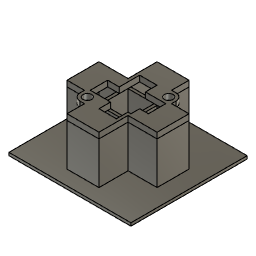
Button+Holder+Rev+3 (Autodesk Fusion 360 design; units mm, degrees)
Autodesk Fusion 360 part; units mm, degrees
note: some values were not read from the file. Set by a fixed rule: which sketch regions a step uses.
sketch "Button Face" plane through (0, 0, 0) normal (0, 0, 1) x (1, 0, 0)
  line L0 (2, 4) -> (44, 4)
  line L1 (44, 4) -> (44, 44)
  line L2 (44, 44) -> (2, 44)
  line L3 (2, 44) -> (2, 4)
  line L4 (7, 30) -> (18, 30)
  line L5 (18, 30) -> (18, 19)
  line L6 (18, 19) -> (7, 19)
  line L7 (7, 19) -> (7, 30)
  line L8 (17, 29) -> (28, 29)
  line L9 (28, 29) -> (28, 40)
  line L10 (28, 40) -> (17, 40)
  line L11 (17, 40) -> (17, 29)
  line L12 (27, 30) -> (38, 30)
  line L13 (38, 30) -> (38, 19)
  line L14 (38, 19) -> (27, 19)
  line L15 (27, 19) -> (27, 30)
  line L16 (17, 20) -> (28, 20)
  line L17 (28, 20) -> (28, 9)
  line L18 (28, 9) -> (17, 9)
  line L19 (17, 9) -> (17, 20)
  line L20 (28, 29) -> (37, 29)
  line L21 (37, 29) -> (37, 20)
  line L22 (37, 20) -> (28, 20)
  line L23 (28, 20) -> (28, 29)
  line L24 (17, 29) -> (8, 29)
  line L25 (8, 29) -> (8, 20)
  line L26 (8, 20) -> (17, 20)
  line L27 (17, 20) -> (17, 29)
  line L28 (18, 19) -> (27, 19)
  line L29 (27, 19) -> (27, 10)
  line L30 (27, 10) -> (18, 10)
  line L31 (18, 10) -> (18, 19)
  line L32 (18, 30) -> (27, 30)
  line L33 (27, 30) -> (27, 39)
  line L34 (27, 39) -> (18, 39)
  line L35 (18, 39) -> (18, 30)
  circle A0 centre (22.5, 14.5) radius 3.6
  circle A1 centre (32.5, 24.5) radius 3.6
  circle A2 centre (22.5, 34.5) radius 3.6
  circle A3 centre (12.5, 24.5) radius 3.6
  circle A4 centre (29.5, 31.5) radius 1.5
  circle A5 centre (29.5, 31.5) radius 2.5
  line L36 (29.5, 34) -> (28, 34)
  line L37 (28, 34) -> (28, 33.5)
  line L38 (28, 33.5) -> (29.5, 33.5)
  line L39 (29.5, 33.5) -> (29.5, 34)
  line L40 (32, 31.5) -> (31.5, 31.5)
  line L41 (31.5, 31.5) -> (31.5, 30)
  line L42 (31.5, 30) -> (32, 30)
  line L43 (32, 30) -> (32, 31.5)
  circle A6 centre (15.5, 17.5) radius 1.5
  circle A7 centre (15.5, 17.5) radius 2.5
  line L44 (15.5, 15) -> (17, 15)
  line L45 (17, 15) -> (17, 15.5)
  line L46 (17, 15.5) -> (15.5, 15.5)
  line L47 (15.5, 15.5) -> (15.5, 15)
  line L48 (13, 17.5) -> (13.5, 17.5)
  line L49 (13.5, 17.5) -> (13.5, 19)
  line L50 (13.5, 19) -> (13, 19)
  line L51 (13, 19) -> (13, 17.5)
  dimension "d3" = 11
  dimension "d4" = 11
  dimension "d5" = 11
  dimension "d6" = 11
  dimension "d7" = 11
  dimension "d8" = 11
  dimension "d9" = 11
  dimension "d10" = 11
  dimension "d11" = 1
  dimension "d12" = 1
  dimension "d13" = 1
  dimension "d14" = 1
  dimension "d15" = 1
  dimension "d16" = 1
  dimension "d17" = 9
  dimension "d18" = 9
  dimension "d19" = 9
  dimension "d20" = 9
  dimension "d21" = 9
  dimension "d22" = 9
  dimension "d23" = 9
  dimension "d24" = 9
  dimension "d25" = 7.2
  dimension "d26" = 4.5
  dimension "d27" = 4.5
  dimension "d28" = 7.2
  dimension "d29" = 7.2
  dimension "d30" = 7.2
  dimension "d31" = 4.5
  dimension "d32" = 4.5
  dimension "d33" = 4.5
  dimension "d34" = 4.5
  dimension "d35" = 4.5
  dimension "d36" = 4.5
  dimension "d38" = 3
  dimension "d39" = 1.5
  dimension "d40" = 1.5
  dimension "d41" = 5
  dimension "d42" = 3
  dimension "d43" = 1.5
  dimension "d44" = 1.5
  dimension "d45" = 5
  constraint horizontal L0
  constraint vertical L1
  constraint horizontal L2
  constraint vertical L3
  constraint horizontal L4
  constraint vertical L5
  constraint horizontal L6
  constraint vertical L7
  constraint horizontal L8
  constraint vertical L9
  constraint horizontal L10
  constraint vertical L11
  constraint horizontal L12
  constraint vertical L13
  constraint horizontal L14
  constraint vertical L15
  constraint horizontal L16
  constraint vertical L17
  constraint horizontal L18
  constraint vertical L19
  constraint horizontal L20
  constraint vertical L21
  constraint horizontal L22
  constraint vertical L23
  constraint horizontal L24
  constraint vertical L25
  constraint horizontal L26
  constraint vertical L27
  constraint horizontal L28
  constraint vertical L29
  constraint horizontal L30
  constraint vertical L31
  constraint horizontal L32
  constraint vertical L33
  constraint horizontal L34
  constraint vertical L35
  constraint concentric A4 A5
  constraint horizontal L36
  constraint vertical L37
  constraint horizontal L38
  constraint vertical L39
  constraint coincident A5 L37.end
  constraint coincident L9 L37.end
  constraint coincident A5 L36.start
  constraint horizontal L40
  constraint vertical L41
  constraint horizontal L42
  constraint vertical L43
  constraint coincident A5 L41.end
  constraint coincident L12 L41.end
  constraint coincident A5 L40.start
  constraint concentric A6 A7
  constraint horizontal L44
  constraint vertical L45
  constraint horizontal L46
  constraint vertical L47
  constraint coincident A7 L45.end
  constraint coincident L19 L45.end
  constraint coincident A7 L44.start
  constraint horizontal L48
  constraint vertical L49
  constraint horizontal L50
  constraint vertical L51
  constraint coincident A7 L49.end
  constraint coincident L6 L49.end
  constraint coincident A7 L48.start
  measures "d3" distance of L4.start L4.end
  measures "d4" distance of L4.start L6.end
  measures "d5" distance of L8.start L8.end
  measures "d6" distance of L8.start L10.end
  measures "d7" distance of L12.start L12.end
  measures "d8" distance of L12.start L14.end
  measures "d9" distance of L16.start L16.end
  measures "d10" distance of L16.start L18.end
  measures "d11" distance of L15 L17
  measures "d12" distance of L14 L16
  measures "d13" distance of L5 L19
  measures "d14" distance of L6 L16
  measures "d15" distance of L9 L15
  measures "d16" distance of L8 L12
  measures "d17" distance of L8.end L20.end
  measures "d18" distance of L8.end L16.end
  measures "d19" distance of L8.start L24.end
  measures "d20" distance of L8.start L16.start
  measures "d21" distance of L5.end L14.end
  measures "d22" distance of L5.end L30.end
  measures "d23" distance of L4.end L12.start
  measures "d24" distance of L4.end L34.end
  measures "d25" diameter of A0
  measures "d26" distance of L31 A0.centre
  measures "d27" distance of L28 A0.centre
  measures "d28" diameter of A1
  measures "d29" diameter of A2
  measures "d30" diameter of A3
  measures "d31" distance of L24 A3.centre
  measures "d32" distance of L25 A3.centre
  measures "d33" distance of L35 A2.centre
  measures "d34" distance of L34 A2.centre
  measures "d35" distance of L23 A1.centre
  measures "d36" distance of L20 A1.centre
  measures "d38" diameter of A4
  measures "d39" distance of L9 A4.centre
  measures "d40" distance of L12 A4.centre
  measures "d41" diameter of A5
  measures "d42" diameter of A6
  measures "d43" distance of L19 A6.centre
  measures "d44" distance of L6 A6.centre
  measures "d45" diameter of A7
extrude "Extrude1" add sketch "Button Face" along normal blind 1 contours L0 L1 L2 L3 | L5 L8 L15 L16 makes body 1 at (36.6667, 10.6667, 0) makes body 2 at (21, 26, 0)
extrude "Extrude2" add sketch "Button Face" along normal blind 15.5 contours L4 L6 L7 L11 L24 L25 L26 A7 L50 | L4 L9 L10 L11 L33 L34 L35 A5 L37 | L4 L5 L8 L11 | L5 L8 L15 L32 | L5 L8 L16 L27 | L6 A7 L50 L51 | L12 L33 A5 | L8 L9 L12 L15 A5 | L5 L6 L16 L19 A7 | L19 L26 A7 | L6 L19 A7 | A7 L48 L49 | L6 L19 A6 A7 L46 L47 L48 L49 | L5 L15 L16 L28 | L8 L15 L16 L23 | L9 L12 A5 | L9 L12 A5 | L9 A5 L36 L37 | L6 L19 A7 | L6 L19 A6 | A7 L46 L47 | L19 A7 L44 L45 | L6 L31 A7 | L14 L15 L16 L17 | L9 L20 A5 | L9 L12 A5 | L9 L12 A4 | L9 L12 A4 A5 L38 L39 L40 L41 | A5 L38 L39 | L6 L19 A7 | L14 L17 L18 L19 L29 L30 L31 A7 L45 | L12 L13 L14 L17 L20 L21 L22 A5 L42 | L12 A5 L42 L43 | A5 L40 L41 bodies 1 2
extrude "Extrude3" add sketch "Button Face" along normal blind 1 contours A6 | A4 bodies 1
extrude "Extrude4" add sketch "Button Face" along normal blind 6.5 contours L32 L33 L34 L35 | L24 L25 L26 L27 | L28 L29 L30 L31 | L20 L21 L22 L23 bodies 1
sketch "Button Back" plane through (0, 0, 15.5) normal (0, 0, 1) x (-1, 0, 0)
  line L0 (-27, -10) -> (-18, -10)
  line L1 (-18, -10) -> (-18, -19)
  line L2 (-18, -19) -> (-27, -19)
  line L3 (-27, -19) -> (-27, -10)
  circle A0 centre (-15.5, -17.5) radius 1.5
  line L4 (-18, -20) -> (-18, -29)
  line L5 (-18, -29) -> (-27, -29)
  line L6 (-27, -29) -> (-27, -20)
  line L7 (-27, -20) -> (-18, -20)
  line L8 (-37, -20) -> (-28, -20)
  line L9 (-28, -20) -> (-28, -29)
  line L10 (-28, -29) -> (-37, -29)
  line L11 (-37, -29) -> (-37, -20)
  circle A1 centre (-29.5, -31.5) radius 1.5
  line L12 (-18, -30) -> (-18, -39)
  line L13 (-18, -39) -> (-27, -39)
  line L14 (-27, -39) -> (-27, -30)
  line L15 (-27, -30) -> (-18, -30)
  line L16 (-17, -29) -> (-17, -20)
  line L17 (-17, -20) -> (-8, -20)
  line L18 (-8, -20) -> (-8, -29)
  line L19 (-8, -29) -> (-17, -29)
  line L20 (-7, -19) -> (-13, -19)
  line L21 (-13, -19) -> (-13, -17.5)
  arc A2 (-13, -17.5) -> (-15.5, -15) centre (-15.5, -17.5) ccw
  line L22 (-15.5, -15) -> (-17, -15)
  line L23 (-17, -15) -> (-17, -9)
  line L24 (-17, -9) -> (-28, -9)
  line L25 (-28, -9) -> (-28, -19)
  line L26 (-28, -19) -> (-38, -19)
  line L27 (-38, -19) -> (-38, -30)
  line L28 (-38, -30) -> (-32, -30)
  line L29 (-32, -30) -> (-32, -31.5)
  arc A3 (-32, -31.5) -> (-29.5, -34) centre (-29.5, -31.5) ccw
  line L30 (-29.5, -34) -> (-28, -34)
  line L31 (-28, -34) -> (-28, -40)
  line L32 (-28, -40) -> (-17, -40)
  line L33 (-17, -40) -> (-17, -30)
  line L34 (-17, -30) -> (-7, -30)
  line L35 (-7, -30) -> (-7, -19)
  line L36 (-8, -29) -> (-17, -29)
  line L37 (-17, -29) -> (-17, -20)
  line L38 (-17, -20) -> (-8, -20)
  line L39 (-8, -20) -> (-8, -29)
  line L40 (-18, -19) -> (-27, -19)
  line L41 (-27, -19) -> (-27, -10)
  line L42 (-27, -10) -> (-18, -10)
  line L43 (-18, -10) -> (-18, -19)
  line L44 (-28, -20) -> (-37, -20)
  line L45 (-37, -20) -> (-37, -29)
  line L46 (-37, -29) -> (-28, -29)
  line L47 (-28, -29) -> (-28, -20)
  line L48 (-27, -30) -> (-18, -30)
  line L49 (-18, -30) -> (-18, -39)
  line L50 (-18, -39) -> (-27, -39)
  line L51 (-27, -39) -> (-27, -30)
  line L52 (-27, -19) -> (-21, -19)
  line L53 (-21, -19) -> (-21, -16)
  line L54 (-21, -16) -> (-27, -16)
  line L55 (-27, -16) -> (-27, -19)
  line L56 (-28, -29) -> (-31, -29)
  line L57 (-31, -29) -> (-31, -23)
  line L58 (-31, -23) -> (-28, -23)
  line L59 (-28, -23) -> (-28, -29)
  line L60 (-18, -30) -> (-24, -30)
  line L61 (-24, -30) -> (-24, -33)
  line L62 (-24, -33) -> (-18, -33)
  line L63 (-18, -33) -> (-18, -30)
  line L64 (-17, -20) -> (-14, -20)
  line L65 (-14, -20) -> (-14, -26)
  line L66 (-14, -26) -> (-17, -26)
  line L67 (-17, -26) -> (-17, -20)
  dimension "d66" = 6
  dimension "d67" = 3
  dimension "d68" = 3
  dimension "d69" = 6
  dimension "d70" = 6
  dimension "d71" = 3
  dimension "d72" = 3
  dimension "d73" = 6
  constraint horizontal L36
  constraint vertical L37
  constraint horizontal L38
  constraint vertical L39
  constraint coincident L16.end L17.start
  constraint coincident L18.end L19.start
  constraint horizontal L40
  constraint vertical L41
  constraint horizontal L42
  constraint vertical L43
  constraint coincident L0.start L3.end
  constraint coincident L1.end L2.start
  constraint horizontal L44
  constraint vertical L45
  constraint horizontal L46
  constraint vertical L47
  constraint coincident L10.end L11.start
  constraint coincident L8.end L9.start
  constraint horizontal L48
  constraint vertical L49
  constraint horizontal L50
  constraint vertical L51
  constraint coincident L12.end L13.start
  constraint coincident L14.end L15.start
  constraint horizontal L52
  constraint vertical L53
  constraint horizontal L54
  constraint vertical L55
  constraint coincident L2.end L3.start
  constraint horizontal L56
  constraint vertical L57
  constraint horizontal L58
  constraint vertical L59
  constraint coincident L9.end L10.start
  constraint horizontal L60
  constraint vertical L61
  constraint horizontal L62
  constraint vertical L63
  constraint coincident L12.start L15.end
  constraint horizontal L64
  constraint vertical L65
  constraint horizontal L66
  constraint vertical L67
  measures "d66" distance of L2.end L52.end
  measures "d67" distance of L2.end L54.end
  measures "d68" distance of L9.end L56.end
  measures "d69" distance of L9.end L58.end
  measures "d70" distance of L12.start L60.end
  measures "d71" distance of L12.start L62.end
  measures "d72" distance of L16.end L64.end
  measures "d73" distance of L16.end L66.end
extrude "Extrude5" add sketch "Button Back" along normal blind 1 separate body contours L0 L1 L2 L3 L40 L41 L42 L43 L53 L54 | L8 L9 L10 L11 L44 L45 L46 L47 L57 L58 | L12 L13 L14 L15 L48 L49 L50 L51 L61 L62 | L16 L17 L18 L19 L36 L37 L38 L39 L65 L66 | L20 L21 A2 L22 L23 L24 L25 L26 L27 L28 L29 A3 L30 L31 L32 L33 L34 L35 makes body 3
sketch "Back Wire" plane through (0, 0, 16.5) normal (0, 0, 1) x (-1, 0, 0)
  line L0 (-17, -26) -> (-17, -20)
  line L1 (-18, -30) -> (-18, -33)
  line L2 (-24, -30) -> (-18, -30)
  circle A0 centre (-15.5, -17.5) radius 1.5
  line L3 (-28, -23) -> (-28, -29)
  circle A1 centre (-29.5, -31.5) radius 1.5
  line L4 (-27, -29) -> (-27, -20)
  line L5 (-27, -20) -> (-18, -20)
  line L6 (-18, -20) -> (-18, -29)
  line L7 (-18, -29) -> (-27, -29)
  line L8 (-27, -19) -> (-27, -16)
  line L9 (-21, -19) -> (-27, -19)
  line L10 (-7, -30) -> (-7, -19)
  line L11 (-7, -19) -> (-13, -19)
  line L12 (-13, -19) -> (-13, -17.5)
  arc A2 (-13, -17.5) -> (-15.5, -15) centre (-15.5, -17.5) ccw
  line L13 (-15.5, -15) -> (-17, -15)
  line L14 (-17, -15) -> (-17, -9)
  line L15 (-17, -9) -> (-28, -9)
  line L16 (-28, -9) -> (-28, -19)
  line L17 (-28, -19) -> (-38, -19)
  line L18 (-38, -19) -> (-38, -30)
  line L19 (-38, -30) -> (-32, -30)
  line L20 (-32, -30) -> (-32, -31.5)
  arc A3 (-32, -31.5) -> (-29.5, -34) centre (-29.5, -31.5) ccw
  line L21 (-29.5, -34) -> (-28, -34)
  line L22 (-28, -34) -> (-28, -40)
  line L23 (-28, -40) -> (-17, -40)
  line L24 (-17, -40) -> (-17, -30)
  line L25 (-17, -30) -> (-7, -30)
  line L26 (-17, -26) -> (-18, -26)
  line L27 (-18, -26) -> (-18, -20)
  line L28 (-18, -20) -> (-17, -20)
  line L29 (-17, -20) -> (-17, -26)
  line L30 (-18, -30) -> (-24, -30)
  line L31 (-24, -30) -> (-24, -29)
  line L32 (-24, -29) -> (-18, -29)
  line L33 (-18, -29) -> (-18, -30)
  line L34 (-27, -19) -> (-21, -19)
  line L35 (-21, -19) -> (-21, -20)
  line L36 (-21, -20) -> (-27, -20)
  line L37 (-27, -20) -> (-27, -19)
  line L38 (-27, -20) -> (-28, -20)
  line L39 (-28, -20) -> (-28, -29)
  line L40 (-28, -29) -> (-27, -29)
  line L41 (-27, -29) -> (-27, -20)
  line L42 (-28, -29) -> (-31, -29)
  line L43 (-17, -20) -> (-14, -20)
  line L44 (-18, -33) -> (-24, -33)
  line L45 (-24, -33) -> (-24, -30)
  line L46 (-27, -16) -> (-21, -16)
  line L47 (-21, -16) -> (-21, -19)
  line L48 (-14, -26) -> (-17, -26)
  line L49 (-14, -20) -> (-14, -26)
  line L50 (-31, -23) -> (-28, -23)
  line L51 (-31, -29) -> (-31, -23)
  constraint horizontal L26
  constraint vertical L27
  constraint horizontal L28
  constraint vertical L29
  constraint coincident L6 L5.end
  constraint coincident L0.start L26.start
  constraint horizontal L30
  constraint vertical L31
  constraint horizontal L32
  constraint vertical L33
  constraint coincident L7 L31.end
  constraint coincident L1.start L2.end
  constraint horizontal L34
  constraint vertical L35
  constraint horizontal L36
  constraint vertical L37
  constraint coincident L5 L35.end
  constraint coincident L8.start L9.end
  constraint horizontal L38
  constraint vertical L39
  constraint horizontal L40
  constraint vertical L41
  constraint coincident L3.end L39.end
  constraint coincident L4.end L5.start
extrude "Extrude6" cut sketch "Back Wire" against normal blind 1 contours L0 L6 L26 L27 L28 L29 | L2 L7 L30 L31 L32 L33 | L5 L9 L34 L35 L36 L37 | L3 L4 L38 L39 L40 L41 bodies 3
copy_body "Body->Comp1" bodies 1 removing the originals makes body 4 in component "Button Holder Face"
copy_body "Body->Comp2" bodies 3 removing the originals makes body 5 in component "Button Holder Back"
extrude "Extrude1'" add 1 faces at (23, 37.6667, 16.5) along direction (0, 0, 1) blind 1 on bodies 5 bodies 5 in component "Button Holder Back"
component "Button Holder Face" placed x (1, 0, 0) y (0, 1, 0) z (0, 0, 1) at (0, 0, 0)
component "Button Holder Back" placed x (1, 0, 0) y (0, 1, 0) z (0, 0, 1) at (0, 0, 0)
equation "d48 = 6.5 mm + 9 mm"
named bodies: "Button Holder Face", "Button Holder Back"
